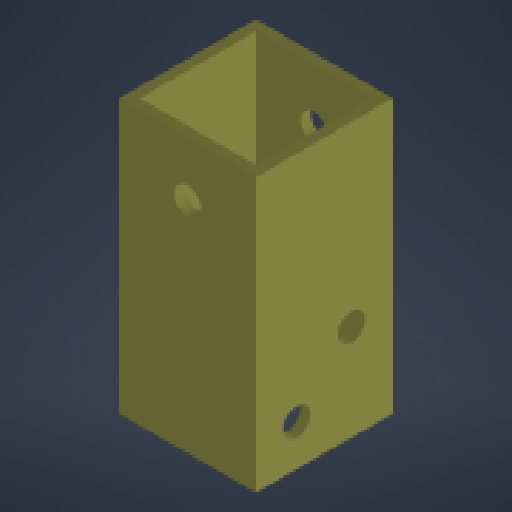
# Autodesk Inventor part: square_box_side_section
Saved by Autodesk Inventor 2024 (Build 280153000, 153)
## iProperties
Created: 2023-04-16
Part Number: square_box_side_section
Material: Типовые
Document SubType Name: Modeling
Designer: user
Density: 1 g/cm^3
Appearance: По умолчанию
Author: user
Autodesk Inventor part; units mm, degrees
ref_plane "YZ Plane" through (0, 0, 0) normal (1, 0, 0) x (0, 1, 0)
ref_plane "XZ Plane" through (0, 0, 0) normal (0, 1, 0) x (-1, 0, 0)
ref_plane "XY Plane" through (0, 0, 0) normal (0, 0, 1) x (1, 0, 0)
ref_plane "РабПлоскость1" through (0, 0, 0) normal (0, 0, 1) x (1, 0, 0)
sketch "Эскиз1" plane through (0, 0, 0) normal (0, 0, 1) x (1, 0, 0)
  line L0 (0, 380) -> (20, 380) projected
  line L1 (20, 380) -> (20, 360) projected
  line L2 (0, 380) -> (0, 360) projected
  line L3 (0, 380) -> (20, 380)
  line L4 (20, 380) -> (20, 360)
  line L5 (20, 360) -> (0, 360)
  line L6 (0, 360) -> (0, 380)
  line L7 (1.5, 378.5) -> (18.5, 378.5)
  line L8 (18.5, 378.5) -> (18.5, 361.5)
  line L9 (18.5, 361.5) -> (1.5, 361.5)
  line L10 (1.5, 361.5) -> (1.5, 378.5)
  point P0 (0, 0)
  point P1 (18.5, 370)
  point P2 (20, 370)
  point P3 (10, 361.5)
  point P4 (10, 360)
  dimension "d0" = 1.5
  constraints: 16 end point, 4 midpoint, 4 parallel, 3 perpendicular, 2 horizontal, 1 horizontal alignment, 1 vertical alignment
  measures "d0" horizontal distance of L2.end L9.end
extrude "Выдавливание1" add sketch "Эскиз1" along normal blind 40
ref_plane "РабПлоскость2" through (-2, 360, -40) normal (-1, 0, 0) x (0, 0, 1)
sketch "Эскиз2" plane through (20, 360, 0) normal (1, 0, 0) x (0, 0, -1)
  circle A0 centre (-14, 14) radius 2 projected
  circle A1 centre (-6, 6) radius 2 projected
  point P0 (0, -360)
extrude "Выдавливание2" cut sketch "Эскиз2" against normal up to surface (22 mm away)
sketch "Эскиз3" plane through (0, 380, 0) normal (0, 1, 0) x (1, 0, 0)
  circle A0 centre (10, -32) radius 2
  line L0 (20, -40) -> (0, -40) projected
  line L1 (20, -20) -> (22, -20) projected
  line L2 (20, 0) -> (20, -40) construction
  line L3 (20, -20) -> (20, -40) construction
  point P0 (0, 0)
  point P1 (10, -40)
  point P2 (20, -30)
  dimension "d5" = 4
  dimension "d8" = 8
  constraints: 2 end point, 2 midpoint, 1 centre point, 1 perpendicular, 1 vertical alignment
  measures "d5" diameter of A0
  measures "d8" vertical distance of L0.start A0.centre
extrude "Выдавливание3" cut sketch "Эскиз3" against normal through all
